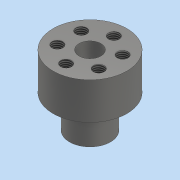
# Autodesk Inventor part: Tuleja zaciskowo rozprężna RCK BK 80 8x15 Clampex
Saved by Autodesk Inventor 2018 (Build 220112000, 112)
## iProperties
Created: 2019-01-25
Part Number: Tuleja zaciskowo rozprężna RCK BK 80 8x15 Clampex
Material: Ogólny
Document SubType Name: Modeling
Designer: Dawid
Density: 1 g/cm^3
Appearance: Anodowana — jasnoszara
Author: Dawid
Autodesk Inventor part; units mm, degrees
ref_plane "YZ Plane" through (0, 0, 0) normal (1, 0, 0) x (0, 1, 0)
ref_plane "XZ Plane" through (0, 0, 0) normal (0, 1, 0) x (-1, 0, 0)
ref_plane "XY Plane" through (0, 0, 0) normal (0, 0, 1) x (1, 0, 0)
sketch "Szkic1" plane through (0, 0, 0) normal (0, 0, 1) x (1, 0, 0)
  circle A0 centre (0, 0) radius 13.5
  dimension "d0" = 27
  constraints: 1 centre point, 1 coincident
  measures "d0" diameter of A0
extrude "Wyciągnięcie proste1" add sketch "Szkic1" along normal blind 25.5
sketch "Szkic2" plane through (0, 0, 0) normal (0, 0, -1) x (-1, 0, 0)
  circle A0 centre (0, 0) radius 7.5
  circle A1 centre (0, 0) radius 13.5 projected
  dimension "d3" = 15
  constraints: 1 centre point, 1 coincident
  measures "d3" diameter of A0
extrude "Wyciągnięcie proste2" cut sketch "Szkic2" against normal blind 12
sketch "Szkic3" plane through (0, 0, 0) normal (0, 0, -1) x (-1, 0, 0)
  circle A0 centre (0, 0) radius 4
  dimension "d6" = 8
  constraints: 1 centre point, 1 coincident
  measures "d6" diameter of A0
extrude "Wyciągnięcie proste3" cut sketch "Szkic3" against normal up to next
sketch "Szkic4" plane through (0, 0, 25.5) normal (0, 0, 1) x (1, 0, 0)
  circle A0 centre (0, 0) radius 4 projected
  circle A1 centre (0, 0) radius 13.5 projected
  line L0 (0, 0) -> (0, 8.75)
  circle A2 centre (0, 8.75) radius 2
  dimension "d11" = 8.75
  dimension "d12" = 4
  constraints: 2 coincident, 2 end point, 1 centre point, 1 vertical
  measures "d11" distance of L0.start L0.end
  measures "d12" diameter of A2
extrude "Wyciągnięcie proste4" cut sketch "Szkic4" against normal blind 12 contours A2
pattern_circular "Szyk kołowy1" count 6 over 360 about axis through (0, 0, 0) along (0, 0, 1) of "Wyciągnięcie proste4"
thread "Gwint1" size "M4x0.7" class "6H" standard "ANSI Metric M Profile" full length
thread "Gwint2" size "M4x0.7" class "6H" standard "ANSI Metric M Profile" full length
thread "Gwint3" size "M4x0.7" class "6H" standard "ANSI Metric M Profile" full length
thread "Gwint4" size "M4x0.7" class "6H" standard "ANSI Metric M Profile" full length
thread "Gwint5" size "M4x0.7" class "6H" standard "ANSI Metric M Profile" full length
thread "Gwint6" size "M4x0.7" class "6H" standard "ANSI Metric M Profile" full length
